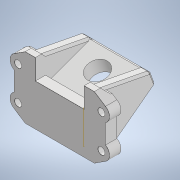
# Autodesk Inventor part: Angle Support Top Anchor
Saved by Autodesk Inventor 2020 (Build 240168000, 168)
## iProperties
Created: 2019-06-01
Part Number: Angle Support Top Anchor
Material: Generic
Document SubType Name: Modeling
Designer: Parker
Density: 1 g/cm^3
Appearance: Default
Author: Parker
Autodesk Inventor part; units mm, degrees
ref_plane "YZ Plane" through (0, 0, 0) normal (1, 0, 0) x (0, 1, 0)
ref_plane "XZ Plane" through (0, 0, 0) normal (0, 1, 0) x (-1, 0, 0)
ref_plane "XY Plane" through (0, 0, 0) normal (0, 0, 1) x (1, 0, 0)
sketch "Sketch1" plane through (0, 0, 0) normal (0, 0, 1) x (1, 0, 0)
  line L0 (22.5, 7.5) -> (-22.5, 7.5)
  line L1 (-22.5, 7.5) -> (-22.5, -7.5)
  line L2 (-22.5, -7.5) -> (22.5, -7.5)
  line L3 (22.5, -7.5) -> (22.5, 7.5)
  point P0 (0, 0)
  dimension "d0" = 45
  dimension "d1" = 15
  dimension "d2" = 22.5
  dimension "d3" = 7.5
  constraints: 8 end point, 2 parallel, 1 horizontal, 1 perpendicular
  measures "d0" distance of L0.start L0.end
  measures "d1" distance of L0.end L1.end
  measures "d2" distance from line of L1 point (0, 0)
  measures "d3" distance from line of L0 point (0, 0)
extrude "Extrusion1" add sketch "Sketch1" along normal blind 5
ref_plane "Work Plane2" through (12, -7.5, 0) normal (1, 0, 0) x (0, 0, -1)
sketch "Sketch3" plane through (12, -7.5, 0) normal (1, 0, 0) x (0, 0, -1)
  line L0 (3.5634, 9.8452) -> (124.385, -322.1095) construction
  line L1 (0, 0) -> (-5, 0) projected
  line L2 (0, 0) -> (18.1105, 6.5917) construction
  line L3 (0, 15) -> (18.1105, 21.5917) construction
  line L4 (-5, 0) -> (-5, 15) projected
  line L5 (0, 7.5) -> (18.4526, 14.2162) construction
  line L6 (0, 11.2246) -> (23, 19.5959)
  line L7 (0, 3.7754) -> (25.3941, 13.0181)
  line L8 (0, 0) -> (0, 15) projected
  line L9 (25.3941, 13.0181) -> (23, 19.5959)
  point P0 (0, 11.2246)
  dimension "d16" = 90
  dimension "d18" = 70
  dimension "d19" = 3.5
  dimension "d20" = 3.5
  dimension "d31" = 23
  constraints: 14 end point, 4 parallel, 2 point on line, 1 coincident, 1 perpendicular
  measures "d16" angle of L0 L2
  measures "d18" angle of L4 L2
  measures "d19" distance between parallel lines of L5 L6
  measures "d20" distance between parallel lines of L5 L7
  measures "d31" horizontal distance of point (0, 11.225) L6.end
extrude "Extrusion2" add sketch "Sketch3" against normal blind 24
sketch "Sketch4" plane through (-12, -3.7246, 0) normal (0, -0.9396926, -0.3420201) x (1, 0, 0)
  line L0 (24, -27.0239) -> (0, -27.0239) projected
  point P0 (12, -1.2739)
  point P1 (12, -17.0239)
  dimension "d32" = 10
  measures "d32" distance from line of L0 point (12, -17.024)
hole "Hole2" at (0, 2.0979, -15.9972) direction (0, 0.9396926, 0.3420201) diameter 10.2 end through all
sketch "Sketch5" plane through (12, -7.5, 0) normal (1, 0, 0) x (0, 0, -1)
  line L0 (-5, 0) -> (-5, 15) projected
  line L1 (-5, 15) -> (-5, 25)
  line L2 (23, 19.5959) -> (0, 11.2246) projected
  line L3 (-5, 25) -> (23, 19.5959)
  line L4 (0, 0) -> (0, 15) projected
  line L5 (0, 15) -> (-5, 15) projected
  line L6 (-5, 0) -> (-5, 15) projected
  line L7 (0, 0) -> (-5, 0) projected
  line L8 (25.3941, 13.0181) -> (23, 19.5959) projected
  line L9 (23, 19.5959) -> (0, 11.2246) projected
  line L10 (0, 3.7754) -> (0, 11.2246) projected
  line L11 (0, 3.7754) -> (25.3941, 13.0181) projected
  line L12 (-5, 0) -> (-5, -10)
  line L13 (-5, -10) -> (25.3941, 13.0181)
  point P0 (-5, 15)
  dimension "d34" = 10
  dimension "d35" = 10
  constraints: 8 end point, 2 vertical, 1 point on line
  measures "d34" distance of L0.end L1.end
  measures "d35" distance of L6.start L12.end
extrude "Extrusion3" add sketch "Sketch5" along normal blind 5 contours L7 L4 L11 L13 L12 | L1 L3 L2 L4 L5 | L4 L2 L8 L11
sketch "Sketch6" plane through (-12, -7.5, 0) normal (-1, 0, 0) x (0, 0, 1)
  line L0 (-23, 19.5959) -> (0, 11.2246) projected
  line L1 (0, 15) -> (0, 11.2246) projected
  line L2 (5, 15) -> (0, 15) projected
  line L3 (5, 25) -> (5, 15) projected
  line L4 (-23, 19.5959) -> (5, 25) projected
  line L5 (-23, 19.5959) -> (-25.3941, 13.0181) projected
  line L6 (-25.3941, 13.0181) -> (0, 3.7754) projected
  line L7 (0, 11.2246) -> (0, 3.7754) projected
  line L8 (0, 11.2246) -> (-23, 19.5959) projected
  line L9 (0, 3.7754) -> (-25.3941, 13.0181) projected
  line L10 (5, -10) -> (-25.3941, 13.0181) projected
  line L11 (5, 0) -> (5, -10) projected
  line L12 (0, 0) -> (5, 0) projected
  line L13 (0, 3.7754) -> (0, 0) projected
  point P0 (0, 7.5)
  point P1 (0, 3.7754)
  point P2 (0, 11.2246)
extrude "Extrusion4" add sketch "Sketch6" along normal blind 5
sketch "Sketch7" plane through (0, 0, 0) normal (0, 0, -1) x (-1, 0, 0)
  line L0 (-17, -7.5) -> (-17, 7.5) projected
  line L1 (-22.5, 7.5) -> (-17, 7.5) projected
  line L2 (-22.5, -7.5) -> (-22.5, 7.5) projected
  line L3 (-17, -7.5) -> (-22.5, -7.5) projected
  line L4 (17, 7.5) -> (17, -7.5) projected
  line L5 (22.5, -7.5) -> (17, -7.5) projected
  line L6 (22.5, 7.5) -> (22.5, -7.5) projected
  line L7 (17, 7.5) -> (22.5, 7.5) projected
  line L8 (-17, 12.0959) -> (-17, 17.5) projected
  line L9 (-22.5, 7.5) -> (-17, 7.5)
  line L10 (-17, 7.5) -> (-17, 17.5)
  line L11 (-17, 17.5) -> (-22.5, 17.5)
  line L12 (-22.5, 17.5) -> (-22.5, 7.5)
  line L13 (12, 17.5) -> (17, 17.5) projected
  line L14 (22.5, 7.5) -> (22.5, -7.5) projected
  line L15 (17, 17.5) -> (22.5, 17.5)
  line L16 (22.5, 17.5) -> (22.5, 7.5)
  line L17 (22.5, 7.5) -> (17, 7.5)
  line L18 (17, 7.5) -> (17, 17.5)
  line L19 (-17, -7.5) -> (-17, -17.5) projected
  line L20 (-22.5, -7.5) -> (-17, -7.5)
  line L21 (-17, -7.5) -> (-17, -17.5)
  line L22 (-17, -17.5) -> (-22.5, -17.5)
  line L23 (-22.5, -17.5) -> (-22.5, -7.5)
  line L24 (22.5, -7.5) -> (17, -7.5) projected
  line L25 (17, 5.5181) -> (17, -17.5) projected
  line L26 (22.5, -7.5) -> (17, -7.5)
  line L27 (17, -7.5) -> (17, -17.5)
  line L28 (17, -17.5) -> (22.5, -17.5)
  line L29 (22.5, -17.5) -> (22.5, -7.5)
  point P0 (0, 0)
  point P1 (17, 7.5)
  point P2 (-17, 7.5)
  constraints: 32 end point, 8 parallel, 4 horizontal, 4 perpendicular
extrude "Extrusion5" add sketch "Sketch7" against normal blind 5 contours L19 L22 L23 L3 | L1 L12 L11 L8 L10 | L18 L15 L16 L7 | L5 L29 L28 L25
sketch "Sketch9" plane through (17, -17.5, 0) normal (-1, 0, 0) x (0, 0, 1)
  line L0 (0, 0) -> (0, 3.7866) projected
  line L1 (0, 10) -> (5, 10) projected
  line L2 (0, 0) -> (5, 0)
  line L3 (5, 0) -> (5, 10)
  line L4 (5, 10) -> (0, 10)
  line L5 (0, 10) -> (0, 0)
  point P0 (0, 17.5)
  constraints: 8 end point, 2 parallel, 1 horizontal, 1 perpendicular
extrude "Extrusion7" add sketch "Sketch9" along normal up to surface (39.5 mm away)
sketch "Sketch8" plane through (0, 0, 0) normal (0, 0, -1) x (-1, 0, 0)
  circle A0 centre (-22.5, -232.1894) radius 1.58 projected
  circle A1 centre (-22.5, -82.1894) radius 1.58 projected
  line L0 (251, -347.9198) -> (246, -342.9198) projected
  line L1 (375, -347.8141) -> (251, -347.9198) projected
  line L2 (379, -343.8141) -> (375, -347.8141) projected
  line L3 (387, -343.8141) -> (379, -343.8141) projected
  line L4 (391, -347.8141) -> (387, -343.8141) projected
  line L5 (411, -347.8141) -> (391, -347.8141) projected
  line L6 (416, -342.8141) -> (411, -347.8141) projected
  line L7 (416, 22.1859) -> (416, -342.8141) projected
  line L8 (411, 27.1859) -> (416, 22.1859) projected
  line L9 (-35, 26.9744) -> (411, 27.1859) projected
  line L10 (-40, 21.9744) -> (-35, 26.9744) projected
  line L11 (-40, -343.0256) -> (-40, 21.9744) projected
  line L12 (-35, -348.0256) -> (-40, -343.0256) projected
  line L13 (-15, -348.0256) -> (-35, -348.0256) projected
  line L14 (-11, -344.0256) -> (-15, -348.0256) projected
  line L15 (-3, -344.0256) -> (-11, -344.0256) projected
  line L16 (1, -348.0256) -> (-3, -344.0256) projected
  line L17 (222, -347.9198) -> (1, -348.0256) projected
  line L18 (227, -342.9198) -> (222, -347.9198) projected
  line L19 (246, -342.9198) -> (227, -342.9198) projected
  circle A2 centre (406, -303.0141) radius 1.5 projected
  circle A3 centre (386, -303.0141) radius 1.5 projected
  circle A4 centre (373.1, -275.0141) radius 1.5 projected
  circle A5 centre (386, 16.9859) radius 1.5 projected
  circle A6 centre (-30, 16.7744) radius 1.5 projected
  circle A7 centre (114.6, -319.8198) radius 2.55 projected
  circle A8 centre (91.4, -319.8198) radius 2.55 projected
  circle A9 centre (77.6, -319.8198) radius 2.55 projected
  circle A10 centre (54.4, -319.8198) radius 2.55 projected
  circle A11 centre (412.3, -161.7141) radius 1.5 projected
  circle A12 centre (412.3, -243.0141) radius 1.5 projected
  circle A13 centre (396, -323.0141) radius 1.5 projected
  circle A14 centre (369, -168.1141) radius 1.5 projected
  circle A15 centre (-30, -303.2256) radius 1.5 projected
  circle A16 centre (-13, -341.0256) radius 1.6 projected
  circle A17 centre (-1, -341.0256) radius 1.6 projected
  circle A18 centre (412.5, -73.5141) radius 1.5 projected
  circle A19 centre (401, -95.0141) radius 1.5 projected
  circle A20 centre (253, -334.9198) radius 1.6 projected
  circle A21 centre (261.4, -319.8198) radius 2.55 projected
  circle A22 centre (220, -334.9198) radius 1.6 projected
  circle A23 centre (143, -334.9198) radius 1.6 projected
  circle A24 centre (284.6, -319.8198) radius 2.55 projected
  circle A25 centre (284.6, -343.0198) radius 2.55 projected
  circle A26 centre (298.4, -319.8198) radius 2.55 projected
  circle A27 centre (298.4, -343.0198) radius 2.55 projected
  circle A28 centre (321.6, -319.8198) radius 2.55 projected
  circle A29 centre (321.6, -343.0198) radius 2.55 projected
  circle A30 centre (220, -343.9198) radius 1.6 projected
  circle A31 centre (261.4, -343.0198) radius 2.55 projected
  circle A32 centre (253, -343.9198) radius 1.6 projected
  circle A33 centre (369.5, -73.5141) radius 1.5 projected
  circle A34 centre (401, -52.0141) radius 1.5 projected
  circle A35 centre (-10, -303.2256) radius 1.5 projected
  circle A36 centre (-20, -323.2256) radius 1.5 projected
  circle A37 centre (369, -243.0141) radius 1.5 projected
  circle A38 centre (373.1, -181.0141) radius 1.5 projected
  circle A39 centre (411.1, -275.0141) radius 1.5 projected
  circle A40 centre (411.1, -181.0141) radius 1.5 projected
  circle A41 centre (143, -343.9198) radius 1.6 projected
  circle A42 centre (54.4, -343.0198) radius 2.55 projected
  circle A43 centre (77.6, -343.0198) radius 2.55 projected
  circle A44 centre (91.4, -343.0198) radius 2.55 projected
  circle A45 centre (114.6, -343.0198) radius 2.55 projected
  circle A46 centre (-10, 16.7744) radius 1.5 projected
  circle A47 centre (406, 16.9859) radius 1.5 projected
  circle A48 centre (376, -340.8141) radius 1.6 projected
  circle A49 centre (390, -340.8141) radius 1.6 projected
  line L20 (366, -296.3141) -> (366, -17.8141) projected
  line L21 (361, -301.3141) -> (366, -296.3141) projected
  line L22 (343, -301.3141) -> (361, -301.3141) projected
  line L23 (333, -311.3141) -> (343, -301.3141) projected
  line L24 (285, -311.4198) -> (333, -311.3141) projected
  line L25 (280, -316.4198) -> (285, -311.4198) projected
  line L26 (266, -316.4198) -> (280, -316.4198) projected
  line L27 (261, -311.4198) -> (266, -316.4198) projected
  line L28 (213, -311.4198) -> (261, -311.4198) projected
  line L29 (193, -331.4198) -> (213, -311.4198) projected
  line L30 (183, -331.4198) -> (193, -331.4198) projected
  line L31 (163, -311.4198) -> (183, -331.4198) projected
  line L32 (115, -311.4198) -> (163, -311.4198) projected
  line L33 (110, -316.4198) -> (115, -311.4198) projected
  line L34 (96, -316.4198) -> (110, -316.4198) projected
  line L35 (91, -311.4198) -> (96, -316.4198) projected
  line L36 (43, -311.5256) -> (91, -311.4198) projected
  line L37 (33, -301.5256) -> (43, -311.5256) projected
  line L38 (15, -301.5256) -> (33, -301.5256) projected
  line L39 (10, -296.5256) -> (15, -301.5256) projected
  line L40 (10, -18.0256) -> (10, -296.5256) projected
  line L41 (15, -13.0256) -> (10, -18.0256) projected
  line L42 (361, -12.8141) -> (15, -13.0256) projected
  line L43 (366, -17.8141) -> (361, -12.8141) projected
  line L44 (10, -29.3001) -> (33, -29.3001)
  line L45 (33, -29.3001) -> (32.99, -13.0146)
  circle A50 centre (20.5, -6.021) radius 1.2295 projected
  circle A51 centre (-20.5, 10.5) radius 1.2295 projected
  circle A52 centre (20.5, 10.5) radius 1.2295 projected
  circle A53 centre (-20.5, -6.021) radius 1.2295 projected
  point P0 (0, 0)
  constraints: 4 end point, 2 point on line, 1 horizontal, 1 perpendicular
extrude "Extrusion6" cut sketch "Sketch8" against normal through all both and the other way through all contours L45 L44 L40 L41 L42
sketch "Sketch10" plane through (-22.5, 17.5, 0) normal (-1, 0, 0) x (0, 0, 1)
  line L0 (5, 0) -> (5, -30.521) projected
  line L1 (5, -30.521) -> (-8.7139, -30.521)
  line L2 (-8.7139, -30.521) -> (-8.7139, -36.1983)
  line L3 (-8.7139, -36.1983) -> (5, -36.1983)
  line L4 (5, -36.1983) -> (5, -30.521)
  point P0 (0, -17.5)
  constraints: 8 end point, 2 parallel, 1 horizontal, 1 perpendicular
extrude "Extrusion8" cut sketch "Sketch10" against normal through all
sketch "Sketch11" plane through (0, 0, 0) normal (0, 0, -1) x (-1, 0, 0)
  line L0 (-22.5, 17.5) -> (-22.5, -13.021) projected
  line L1 (22.5, -13.021) -> (22.5, 17.5) projected
  line L2 (-22.5, -13.021) -> (-17, -13.021) projected
  line L3 (17, -13.021) -> (22.5, -13.021) projected
  line L4 (22.5, 17.5) -> (17, 17.5) projected
  line L5 (-17, 17.5) -> (-22.5, 17.5) projected
  point P0 (0, 0)
  point P1 (-20.5, -6)
  point P2 (20.5, -6)
  point P3 (20.5, 10.5)
  point P4 (-20.5, 10.5)
  dimension "d48" = 2
  dimension "d49" = 2
  dimension "d50" = 2
  dimension "d51" = 2
  dimension "d61" = 7
  dimension "d62" = 7
  dimension "d84" = 16.5
  dimension "d85" = 16.5
  measures "d48" distance from line of L0 point (-20.5, 10.5)
  measures "d49" distance from line of L0 point (-20.5, -6)
  measures "d50" distance from line of L1 point (20.5, -6)
  measures "d51" distance from line of L1 point (20.5, 10.5)
  measures "d61" distance from line of L4 point (20.5, 10.5)
  measures "d62" distance from line of L5 point (-20.5, 10.5)
  measures "d84" distance of point (-20.5, 10.5) point (-20.5, -6)
  measures "d85" distance of point (20.5, 10.5) point (20.5, -6)
hole "Hole3" at (20.5, -6, 0) at (-20.5, -6, 0) at (-20.5, 10.5, 0) at (20.5, 10.5, 0) direction (0, 0, 1) diameter 3.4 end through all clearance for "Flat Head Machine Screw" size "M3" standard "Ansi Metric M Profile"
sketch "Sketch12" plane through (0, 0, 0) normal (0, 0, -1) x (-1, 0, 0)
  circle A0 centre (-20.5, 10.5) radius 1.7 projected
  circle A1 centre (-20.5, 10.5) radius 4
  circle A2 centre (-20.5, -6) radius 1.7 projected
  circle A3 centre (-20.5, -6) radius 4
  circle A4 centre (20.5, -6) radius 1.7 projected
  circle A5 centre (20.5, -6) radius 4
  circle A6 centre (20.5, 10.5) radius 1.7 projected
  circle A7 centre (20.5, 10.5) radius 4
  point P0 (0, 0)
  dimension "d63" = 8
  dimension "d64" = 8
  dimension "d65" = 8
  dimension "d66" = 8
  constraints: 4 centre point, 4 coincident
  measures "d63" diameter of A1
  measures "d64" diameter of A3
  measures "d65" diameter of A5
  measures "d66" diameter of A7
extrude "Extrusion9" add sketch "Sketch12" against normal up to surface (5 mm away)
sketch "Sketch13" plane through (0, 0, 0) normal (0, 0, -1) x (-1, 0, 0)
  line L0 (-22.5, 13.9641) -> (-22.5, 17.5) projected
  line L1 (-12, 17.5) -> (-17, 17.5) projected
  line L2 (-22.5, 13.9641) -> (-17, 17.5)
  line L3 (12, 17.5) -> (17, 17.5) projected
  line L4 (22.5, 17.5) -> (22.5, 13.9641) projected
  line L5 (17, 17.5) -> (22.5, 13.9641)
  line L6 (17, 5.5181) -> (17, -13.021) projected
  line L7 (22.5, -13.021) -> (22.5, -9.4641) projected
  line L8 (17, -13.021) -> (22.5, -9.4641)
  line L9 (-22.5, -13.021) -> (-22.5, -9.4641) projected
  line L10 (-22.5, -9.4641) -> (-17, -13.021)
  line L11 (22.5, -13.021) -> (-22.5, -13.021) projected
  line L12 (-17, 17.5) -> (-22.5, 17.5) projected
  line L13 (22.5, 17.5) -> (17, 17.5) projected
  point P0 (0, 0)
  constraints: 8 end point, 1 point on line
extrude "Extrusion10" cut sketch "Sketch13" against normal blind 10
sketch "Sketch14" plane through (0, 0, 0) normal (0, 0, -1) x (-1, 0, 0)
  line L0 (-12, 17.5) -> (-17, 17.5) projected
  line L1 (-12, 17.5) -> (-12, 7.5) projected
  line L2 (-17, 17.5) -> (-12, 17.5)
  line L3 (-12, 17.5) -> (-12, 12.0694)
  line L4 (-12, 12.0694) -> (-17, 12.0694)
  line L5 (-17, 12.0694) -> (-17, 17.5)
  line L6 (12, 7.5) -> (12, 17.5) projected
  line L7 (17, -13.021) -> (17, 16.535) projected
  line L8 (12, 17.5) -> (17, 17.5)
  line L9 (17, 17.5) -> (17, 12.0694)
  line L10 (17, 12.0694) -> (12, 12.0694)
  line L11 (12, 12.0694) -> (12, 17.5)
  point P0 (0, 0)
  constraints: 16 end point, 4 parallel, 3 point on line, 2 horizontal, 2 perpendicular
extrude "Extrusion11" add sketch "Sketch14" against normal up to surface (5 mm away)
chamfer "Chamfer1" distance 2 angle 45 2 edges at (-14.5, 17.5, 0) (14.5, 17.5, 0)
chamfer "Chamfer2" distance 0.05 angle 45 20 edges at (-22.5, 2.25, 5) (-24.5, 10.5, 5) (-19.75, 15.7321, 5) (-14.5, 17.5, 5) (-12, 12.5, 5) (0, 7.5, 5) (12, 12.5, 5) (14.5, 17.5, 5) (19.75, 15.7321, 5) (24.5, 10.5, 5) (22.5, 2.25, 5) (24.5, -6, 5) (19.75, -11.2426, 5) (0, -13.021, 5) (-19.75, -11.2426, 5) (-24.5, -6, 5) (-20.5, -7.7, 5) (-20.5, 8.8, 5) (20.5, -7.7, 5) (20.5, 8.8, 5)
chamfer "Chamfer3" distance 1 angle 45 18 edges at (0, 5.5181, -25.3941) (0, 12.0959, -23) (-14.5, 12.0959, -23) (14.5, 12.0959, -23) (14.5, 5.5181, -25.3941) (-14.5, 5.5181, -25.3941) (-17, 8.807, -24.1971) (17, 8.807, -24.1971) (-12, -3.7515, -13.1542) (-17, -3.7515, -13.1542) (17, -3.7515, -13.1542) (12, -3.7515, -13.1542) (-17, 14.4392, -10.8587) (-12, 14.4392, -10.8587) (12, 14.4392, -10.8587) (17, 14.4392, -10.8587) (0, 3.7246, 0) (0, -3.7246, 0)
sketch "Sketch15" plane through (0, 0, 0) normal (0, 0, -1) x (-1, 0, 0)
  circle A0 centre (-20.5, -6) radius 1.7 projected
  circle A1 centre (-20.5, 10.5) radius 1.7 projected
  line L0 (-20.1109, 15.5) -> (-17, 15.5) projected
  line L1 (-20.1109, 15.5) -> (-22.5, 13.9641) projected
  arc A2 (-22.5, 13.9641) -> (-22.5, 7.0359) centre (-20.5, 10.5) ccw projected
  line L2 (-22.5, 7.0359) -> (-22.5, -2.5359) projected
  arc A3 (-22.5, -2.5359) -> (-22.5, -9.4641) centre (-20.5, -6) ccw projected
  line L3 (-22.5, -9.4641) -> (-17, -13.021) projected
  line L4 (-17, -13.021) -> (-16.552, -13.021) projected
  line L5 (-17, -12.459) -> (-16.552, -13.021) projected
  line L6 (-17, -12.459) -> (-17, 15.5) projected
  line L7 (17, 15.5) -> (20.1109, 15.5) projected
  line L8 (17, -12.459) -> (17, 15.5) projected
  line L9 (17, -12.459) -> (16.552, -13.021) projected
  line L10 (16.552, -13.021) -> (17, -13.021) projected
  line L11 (17, -13.021) -> (22.5, -9.4641) projected
  arc A4 (22.5, -9.4641) -> (22.5, -2.5359) centre (20.5, -6) ccw projected
  line L12 (22.5, -2.5359) -> (22.5, 7.0359) projected
  arc A5 (22.5, 7.0359) -> (22.5, 13.9641) centre (20.5, 10.5) ccw projected
  line L13 (22.5, 13.9641) -> (20.1109, 15.5) projected
  circle A6 centre (20.5, -6) radius 1.7 projected
  circle A7 centre (20.5, 10.5) radius 1.7 projected
  point P0 (0, 0)
extrude "Extrusion12" add sketch "Sketch15" along normal blind 0.65
body "Solid1"
